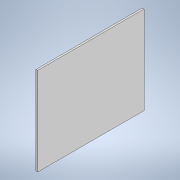
# Autodesk Inventor part: TorraumHinten
Saved by Autodesk Inventor 2021 (Build 250183000, 183)
## iProperties
Created: 2022-02-22
Part Number: TorraumHinten
Material: Generisch
Document SubType Name: Modeling
Designer: valen
Density: 1 g/cm^3
Appearance: Vorgabe
Author: valen
Autodesk Inventor part; units mm, degrees
ref_plane "YZ Plane" through (0, 0, 0) normal (1, 0, 0) x (0, 1, 0)
ref_plane "XZ Plane" through (0, 0, 0) normal (0, 1, 0) x (-1, 0, 0)
ref_plane "XY Plane" through (0, 0, 0) normal (0, 0, 1) x (1, 0, 0)
sketch "Skizze1" plane through (0, 0, 0) normal (1, 0, 0) x (0, 1, 0)
  line L0 (0, 0) -> (192, 0)
  line L1 (192, 0) -> (192, -232)
  line L2 (192, -232) -> (0, -232)
  line L3 (0, -232) -> (0, 0)
  dimension "d0" = 232
  dimension "d1" = 192
  constraints: 8 end point, 2 parallel, 1 horizontal, 1 perpendicular
  measures "d0" distance between parallel lines of L2 L0
  measures "d1" distance between parallel lines of L1 L3
extrude "Extrusion1" add sketch "Skizze1" along normal blind 4
